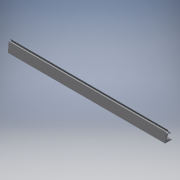
# Autodesk Inventor part: juncao controle tela
Saved by Autodesk Inventor 2016 (Build 200138000, 138)
## iProperties
Created: 2017-06-28
Part Number: juncao controle tela
Material: Genérico
Document SubType Name: Modeling
Designer: Fabio
Density: 1 g/cm^3
Appearance: Padrão
Author: Fabio
Autodesk Inventor part; units mm, degrees
ref_plane "YZ Plane" through (0, 0, 0) normal (1, 0, 0) x (0, 1, 0)
ref_plane "XZ Plane" through (0, 0, 0) normal (0, 1, 0) x (-1, 0, 0)
ref_plane "XY Plane" through (0, 0, 0) normal (0, 0, 1) x (1, 0, 0)
sketch "Esboço1" plane through (0, 0, 0) normal (1, 0, 0) x (0, 1, 0)
  line L0 (0.4443, 5.6274) -> (-0.9413, 9.5119)
  line L1 (0.4443, 5.6274) -> (-3.3612, 4.0485)
  line L2 (-3.3612, 4.0485) -> (-5.5175, 9.2458)
  line L3 (-5.5175, 9.2458) -> (-5.7078, 6.9431)
  line L4 (-7.3945, -13.4652) -> (7.0591, -13.4652)
  line L5 (7.0591, -13.4652) -> (-5.1461, -7.0903)
  line L6 (-5.1461, -7.0903) -> (0.4923, 3.7048)
  line L7 (0.4923, 3.7048) -> (9.7416, -1.1262)
  arc A0 (-0.9413, 9.5119) -> (9.7416, -1.1262) centre (21.579, 21.4439) ccw
  line L8 (-5.7078, 6.9431) -> (-7.3945, -13.4652)
  point P0 (-0.6447, 8.6807)
  constraints: 18 end point, 3 perpendicular, 2 point on circle, 2 point on line, 1 centre point, 1 horizontal
extrude "Extrusão1" add sketch "Esboço1" along normal blind 165
